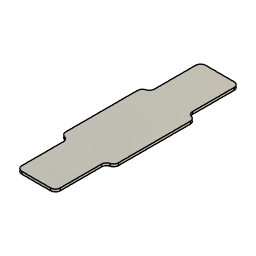
Base (Autodesk Fusion 360 design; units mm, degrees)
Autodesk Fusion 360 part; units mm, degrees
sketch "Sketch1" plane through (0, 0, 0) normal (0, 0, 1) x (1, 0, 0)
  line L0 (54.5, -188.5) -> (-54.5, -188.5)
  line L1 (-54.5, -188.5) -> (-54.5, 188.5)
  line L2 (-54.5, 188.5) -> (54.5, 188.5)
  line L3 (54.5, 188.5) -> (54.5, -188.5)
  line L4 (54.5, -188.5) -> (-54.5, 188.5) construction
  line L5 (-54.5, -188.5) -> (54.5, 188.5) construction
  line L6 (-54.5, 153.5) -> (-39.5, 153.5)
  line L7 (-39.5, 153.5) -> (-39.5, 83.5)
  line L8 (-39.5, 83.5) -> (-54.5, 83.5)
  line L9 (-54.5, 83.5) -> (-54.5, 153.5)
  line L10 (-54.5, -153.5) -> (-39.5, -153.5)
  line L11 (-39.5, -153.5) -> (-39.5, -83.5)
  line L12 (-39.5, -83.5) -> (-54.5, -83.5)
  line L13 (-54.5, -83.5) -> (-54.5, -153.5)
  line L14 (54.5, -153.5) -> (39.5, -153.5)
  line L15 (39.5, -153.5) -> (39.5, -83.5)
  line L16 (39.5, -83.5) -> (54.5, -83.5)
  line L17 (54.5, -83.5) -> (54.5, -153.5)
  line L18 (54.5, 153.5) -> (39.5, 153.5)
  line L19 (39.5, 153.5) -> (39.5, 83.5)
  line L20 (39.5, 83.5) -> (54.5, 83.5)
  line L21 (54.5, 83.5) -> (54.5, 153.5)
  line L22 (-39.5, -153.5) -> (-39.5, -188.5)
  line L23 (39.5, -153.5) -> (39.5, -188.5)
  line L24 (-39.5, 153.5) -> (-39.5, 188.5)
  line L25 (39.5, 153.5) -> (39.5, 188.5)
  dimension "d1" = 109
  dimension "d2" = 377
  dimension "d3" = 15
  dimension "d4" = 70
  dimension "d5" = 15
  dimension "d6" = 70
  dimension "d7" = 35
  dimension "d8" = 35
  dimension "d9" = 15
  dimension "d10" = 70
  dimension "d11" = 15
  dimension "d12" = 70
  constraint horizontal L0
  constraint perpendicular L0 L1
  constraint parallel L0 L2
  constraint parallel L1 L3
  constraint coincident L4 origin
  constraint coincident L5 origin
  constraint horizontal L6
  constraint vertical L7
  constraint horizontal L8
  constraint vertical L9
  constraint coincident L1 L6.start
  constraint horizontal L10
  constraint vertical L11
  constraint horizontal L12
  constraint vertical L13
  constraint coincident L1 L10.start
  constraint horizontal L14
  constraint vertical L15
  constraint horizontal L16
  constraint vertical L17
  constraint coincident L3 L14.start
  constraint horizontal L18
  constraint vertical L19
  constraint horizontal L20
  constraint vertical L21
  constraint coincident L3 L18.start
  constraint coincident L0 L22.end
  constraint perpendicular L0 L22
  constraint coincident L0 L23.end
  constraint perpendicular L0 L23
  constraint coincident L2 L24.end
  constraint perpendicular L2 L24
  constraint coincident L2 L25.end
  constraint perpendicular L2 L25
  measures "d1" distance of L1.end L2.end
  measures "d2" distance of L0.end L1.end
  measures "d3" distance of L6.start L6.end
  measures "d4" distance of L6.start L8.end
  measures "d5" distance of L10.start L10.end
  measures "d6" distance of L10.start L12.end
  measures "d7" distance of L2 L6.start
  measures "d8" distance of L0 L10.end
  measures "d9" distance of L14.start L14.end
  measures "d10" distance of L14.start L16.end
  measures "d11" distance of L18.start L18.end
  measures "d12" distance of L18.start L20.end
extrude "Extrude1" add sketch "Sketch1" along normal blind 5 contours L0 L1 L2 L3 L7 L8 L11 L12 L15 L16 L19 L20 L22 L23 L24 L25
fillet "Fillet1" radius 10 12 edges at (54.5, 83.5, 2.5) (39.5, 83.5, 2.5) (39.5, 188.5, 2.5) (-39.5, 188.5, 2.5) (-39.5, 83.5, 2.5) (-54.5, 83.5, 2.5) (-54.5, -83.5, 2.5) (-39.5, -83.5, 2.5) (-39.5, -188.5, 2.5) (39.5, -188.5, 2.5) (39.5, -83.5, 2.5) (54.5, -83.5, 2.5)
